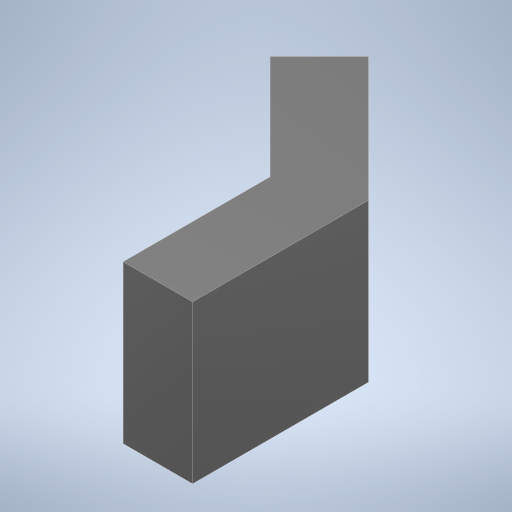
# Autodesk Inventor part: PXCorner
Saved by Autodesk Inventor 2023 (Build 270158000, 158)
## iProperties
Created: 2023-10-08
Part Number: PXCorner
Material: Generic
Document SubType Name: Modeling
Designer: adamarnold
Density: 1 g/cm^3
Appearance: Smooth - Black
Author: adamarnold
Autodesk Inventor part; units mm, degrees
ref_plane "YZ Plane" through (0, 0, 0) normal (1, 0, 0) x (0, 1, 0)
ref_plane "XZ Plane" through (0, 0, 0) normal (0, 1, 0) x (-1, 0, 0)
ref_plane "XY Plane" through (0, 0, 0) normal (0, 0, 1) x (1, 0, 0)
sketch "Sketch1" plane through (0, 0, 0) normal (0, 1, 0) x (-1, 0, 0)
  line L0 (0, 0) -> (0, 50.8)
  line L1 (0, 50.8) -> (20.066, 50.8)
  line L2 (20.066, 50.8) -> (20.066, 8.3116)
  line L3 (0, 0) -> (35.921, -35.921)
  line L4 (0, 0) -> (50.8, 0) construction
  line L5 (35.921, -35.921) -> (50.1098, -21.7322)
  line L6 (35.921, -35.921) -> (55.987, -35.921) construction
  line L7 (50.1098, -21.7322) -> (20.066, 8.3116)
  dimension "d0" = 50.8
  dimension "d1" = 50.8
  dimension "d2" = 45
  dimension "d3" = 20.066
  dimension "d4" = 20.066
  dimension "d5" = 45
  constraints: 16 end point, 3 perpendicular, 2 equal length, 2 horizontal, 1 vertical
  measures "d0" distance of L0.start L0.end
  measures "d1" distance of L0.start L3.end
  measures "d2" angle of L3 L4
  measures "d3" distance of L0.end L1.end
  measures "d4" distance of L3.end L5.end
  measures "d5" angle of L6 L5
extrude "Extrusion1" add sketch "Sketch1" along normal blind 45.466
body "Solid1"
